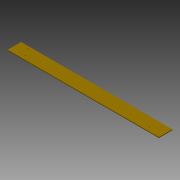
# Autodesk Inventor part: X Rail
Saved by Autodesk Inventor 2013 (Build 170138000, 138)
## iProperties
Created: 2017-01-25
Part Number: X Rail
Material: Generic
Document SubType Name: Modeling
Designer: Herman de Vries
Density: 1 g/cm^3
Author: Herman de Vries
Autodesk Inventor part; units mm, degrees
ref_plane "YZ Plane" through (0, 0, 0) normal (1, 0, 0) x (0, 1, 0)
ref_plane "XZ Plane" through (0, 0, 0) normal (0, 1, 0) x (-1, 0, 0)
ref_plane "XY Plane" through (0, 0, 0) normal (0, 0, 1) x (1, 0, 0)
sketch "Sketch1" plane through (0, 0, 0) normal (1, 0, 0) x (0, 1, 0)
  line L0 (0, 0) -> (50, 0)
  line L1 (50, 0) -> (50, 3)
  line L2 (50, 3) -> (0, 3)
  line L3 (0, 3) -> (0, 0)
  dimension "d0" = 50
  dimension "d1" = 3
  constraints: 8 end point, 2 parallel, 1 horizontal, 1 perpendicular
  measures "d0" distance of L2.end L1.end
  measures "d1" distance of L1.end L0.end
extrude "Extrusion1" add sketch "Sketch1" along normal blind 560
sketch "Sketch2" plane through (0, 0, 3) normal (0, 0, 1) x (1, 0, 0)
  circle A0 centre (35, 40) radius 1.5
  circle A1 centre (51, 15) radius 1.5
  line L0 (0, 0) -> (560, 0) projected
  line L1 (0, 50) -> (560, 50) projected
  line L2 (0, 50) -> (0, 0) projected
  circle A2 centre (530, 40) radius 1.5
  line L3 (560, 50) -> (560, 0) projected
  circle A3 centre (510, 15) radius 1.5
  point P0 (560, 25)
  dimension "d4" = 3
  dimension "d5" = 3
  dimension "d9" = 3
  dimension "d12" = 16
  dimension "d13" = 35
  dimension "d14" = 25
  dimension "d15" = 10
  dimension "d16" = 3
  dimension "d17" = 30
  dimension "d18" = 20
  dimension "d19" = 10
  dimension "d20" = 25
  constraints: 4 centre point, 1 midpoint
  measures "d4" diameter of A0
  measures "d5" diameter of A1
  measures "d9" diameter of A2
  measures "d12" horizontal distance of A1.centre A0.centre
  measures "d13" distance from line of L2 A0.centre
  measures "d14" vertical distance of A1.centre A0.centre
  measures "d15" distance from line of A0.centre L1
  measures "d16" diameter of A3
  measures "d17" distance from line of L3 A2.centre
  measures "d18" horizontal distance of A2.centre A3.centre
  measures "d19" distance from line of L1 A2.centre
  measures "d20" vertical distance of A3.centre A2.centre
extrude "Extrusion2" cut sketch "Sketch2" against normal blind 10 contours A0 | A1 | A2 | A3
equation "\"d5\" = d4"
equation "\"d9\" = d4"
equation "\"d16\" = d9"
equation "\"d19\" = d15"
equation "\"d20\" = d14"
body "Solid1"
